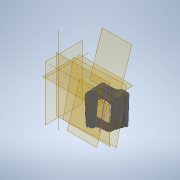
# Autodesk Inventor part: WaveRunnerFootPedal
Saved by Autodesk Inventor 2021 (Build 250183000, 183)
## iProperties
Created: 2021-02-10
Part Number: WaveRunnerFootPedal
Material: Generic
Document SubType Name: Modeling
Designer: Viktor
Density: 1 g/cm^3
Appearance: Default
Author: Viktor
Autodesk Inventor part; units mm, degrees
ref_plane "Work Plane2" through (0, -64.8936, -199.7219) normal (0, 0.309017, 0.9510565) x (1, 0, 0)
ref_plane "Work Plane1" through (0, 0, 0) normal (0, 0.309017, 0.9510565) x (1, 0, 0)
sketch "Sketch1" plane through (0, -64.8936, -199.7219) normal (0, 0.309017, 0.9510565) x (1, 0, 0)
  line L0 (397, 0) -> (438, -432)
  point P0 (0, 0)
  constraints: 2 end point
ref_plane "Work Plane3" through (397, -64.8936, -199.7219) normal (-0.1213242, 0.2957626, 0.9475257) x (0.0944828, -0.946802, 0.3076346)
sketch "Sketch2" plane through (397, -64.8936, -199.7219) normal (-0.1213242, 0.2957626, 0.9475257) x (0.0944828, -0.946802, 0.3076346)
  line L0 (166, 115) -> (324.3894, 96.0131)
  line L1 (324.3894, 96.0131) -> (321, -76)
  line L2 (321, -76) -> (162, -88)
  line L3 (162, -88) -> (166, 115)
  point P0 (-37.5097, -366.6855)
  constraints: 8 end point, 1 parallel
extrude "Extrusion1" add sketch "Sketch2" against normal blind 67.25
body "Solid1"
